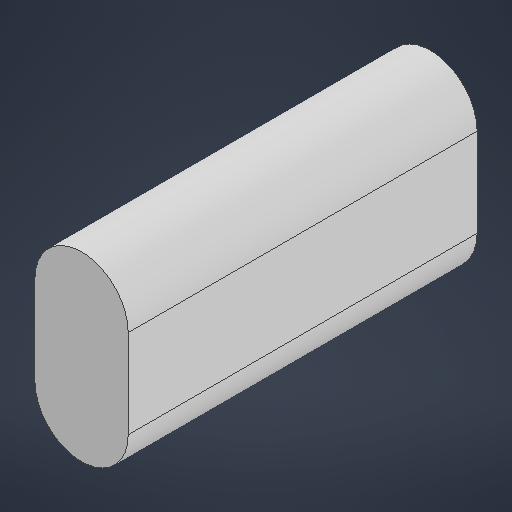
# Autodesk Inventor part: 电池
Saved by Autodesk Inventor 2025 (Build 290162000, 162)
## iProperties
Created: 2026-03-02
Part Number: 电池
Material: 常规
Document SubType Name: Modeling
Designer: XH
Density: 1 g/cm^3
Appearance: 默认
Author: XH
Autodesk Inventor part; units mm, degrees
ref_plane "YZ Plane" through (0, 0, 0) normal (1, 0, 0) x (0, 1, 0)
ref_plane "XZ Plane" through (0, 0, 0) normal (0, 1, 0) x (-1, 0, 0)
ref_plane "XY Plane" through (0, 0, 0) normal (0, 0, 1) x (1, 0, 0)
sketch "草图1" plane through (0, 0, 0) normal (0, 0, 1) x (1, 0, 0)
  line L0 (0, 0) -> (0, -18) construction
  line L1 (-9.5, 0) -> (-9.5, -18)
  line L2 (9.5, -18) -> (9.5, 0)
  arc A0 (9.5, 0) -> (-9.5, 0) centre (0, 0) ccw
  arc A1 (-9.5, -18) -> (9.5, -18) centre (0, -18) ccw
  point P0 (0, -9)
  point P1 (0, 9.5)
  point P2 (0, -27.5)
  dimension "d0" = 19
  dimension "d1" = 37
  constraints: 8 end point, 6 point on circle, 4 tangent, 2 centre point, 1 midpoint, 1 parallel, 1 vertical
  measures "d0" distance between parallel lines of L1 L2
  measures "d1" distance of point (0, 9.5) point (0, -27.5)
extrude "拉伸1" add sketch "草图1" along normal blind 71
